Autodesk Inventor part; units mm, degrees
(part 6 of 15)
  arc A2446 (57.485, 40.2522) -> (57.485, 40.3538) centre (57.485, 40.303) ccw
  line L1082 (56.215, 40.303) -> (56.215, 43.097)
  arc A2447 (56.2658, 43.097) -> (56.1642, 43.097) centre (56.215, 43.097) ccw
  arc A2448 (56.1642, 40.303) -> (56.2658, 40.303) centre (56.215, 40.303) ccw
  line L1083 (56.215, 43.097) -> (57.485, 43.097)
  arc A2449 (57.485, 43.0462) -> (57.485, 43.1478) centre (57.485, 43.097) ccw
  arc A2450 (56.215, 43.1478) -> (56.215, 43.0462) centre (56.215, 43.097) ccw
  line L1084 (-14.55, 7.3) -> (-13.46, 7.3)
  line L1085 (59.642, 47.084) -> (59.642, 49.116)
  arc A2451 (59.6928, 49.116) -> (59.5912, 49.116) centre (59.642, 49.116) ccw
  arc A2452 (59.5912, 47.084) -> (59.6928, 47.084) centre (59.642, 47.084) ccw
  line L1086 (59.642, 49.116) -> (60.658, 49.116)
  arc A2453 (60.658, 49.0652) -> (60.658, 49.1668) centre (60.658, 49.116) ccw
  arc A2454 (59.642, 49.1668) -> (59.642, 49.0652) centre (59.642, 49.116) ccw
  line L1087 (60.658, 49.116) -> (60.658, 47.084)
  arc A2455 (60.6072, 47.084) -> (60.7088, 47.084) centre (60.658, 47.084) ccw
  arc A2456 (60.7088, 49.116) -> (60.6072, 49.116) centre (60.658, 49.116) ccw
  line L1088 (60.658, 47.084) -> (59.642, 47.084)
  arc A2457 (59.642, 47.1348) -> (59.642, 47.0332) centre (59.642, 47.084) ccw
  arc A2458 (60.658, 47.0332) -> (60.658, 47.1348) centre (60.658, 47.084) ccw
  arc A2459 (-13.46, 7.275) -> (-13.46, 7.325) centre (-13.46, 7.3) ccw
  line L1089 (52.658, 51.116) -> (52.658, 49.084)
  arc A2460 (52.6072, 49.084) -> (52.7088, 49.084) centre (52.658, 49.084) ccw
  arc A2461 (52.7088, 51.116) -> (52.6072, 51.116) centre (52.658, 51.116) ccw
  line L1090 (52.658, 49.084) -> (51.642, 49.084)
  arc A2462 (51.642, 49.1348) -> (51.642, 49.0332) centre (51.642, 49.084) ccw
  arc A2463 (52.658, 49.0332) -> (52.658, 49.1348) centre (52.658, 49.084) ccw
  line L1091 (51.642, 49.084) -> (51.642, 51.116)
  arc A2464 (51.6928, 51.116) -> (51.5912, 51.116) centre (51.642, 51.116) ccw
  arc A2465 (51.5912, 49.084) -> (51.6928, 49.084) centre (51.642, 49.084) ccw
  line L1092 (51.642, 51.116) -> (52.658, 51.116)
  arc A2466 (52.658, 51.0652) -> (52.658, 51.1668) centre (52.658, 51.116) ccw
  arc A2467 (51.642, 51.1668) -> (51.642, 51.0652) centre (51.642, 51.116) ccw
  arc A2468 (-14.55, 7.325) -> (-14.55, 7.275) centre (-14.55, 7.3) ccw
  line L1093 (46.293, 49.3892) -> (46.293, 44.4108)
  arc A2469 (46.2422, 44.4108) -> (46.3438, 44.4108) centre (46.293, 44.4108) ccw
  arc A2470 (46.3438, 49.3892) -> (46.2422, 49.3892) centre (46.293, 49.3892) ccw
  line L1094 (46.293, 44.4108) -> (44.007, 44.4108)
  arc A2471 (44.007, 44.4616) -> (44.007, 44.36) centre (44.007, 44.4108) ccw
  arc A2472 (46.293, 44.36) -> (46.293, 44.4616) centre (46.293, 44.4108) ccw
  line L1095 (44.007, 44.4108) -> (44.007, 49.3892)
  arc A2473 (44.0578, 49.3892) -> (43.9562, 49.3892) centre (44.007, 49.3892) ccw
  arc A2474 (43.9562, 44.4108) -> (44.0578, 44.4108) centre (44.007, 44.4108) ccw
  line L1096 (44.007, 49.3892) -> (46.293, 49.3892)
  arc A2475 (46.293, 49.3384) -> (46.293, 49.44) centre (46.293, 49.3892) ccw
  arc A2476 (44.007, 49.44) -> (44.007, 49.3384) centre (44.007, 49.3892) ccw
  line L1097 (-14.75, 4.1) -> (-14.75, 7.3)
  line L1098 (49.634, 46.108) -> (51.666, 46.108)
  arc A2477 (51.666, 46.0572) -> (51.666, 46.1588) centre (51.666, 46.108) ccw
  arc A2478 (49.634, 46.1588) -> (49.634, 46.0572) centre (49.634, 46.108) ccw
  line L1099 (51.666, 46.108) -> (51.666, 45.092)
  arc A2479 (51.6152, 45.092) -> (51.7168, 45.092) centre (51.666, 45.092) ccw
  arc A2480 (51.7168, 46.108) -> (51.6152, 46.108) centre (51.666, 46.108) ccw
  line L1100 (51.666, 45.092) -> (49.634, 45.092)
  arc A2481 (49.634, 45.1428) -> (49.634, 45.0412) centre (49.634, 45.092) ccw
  arc A2482 (51.666, 45.0412) -> (51.666, 45.1428) centre (51.666, 45.092) ccw
  line L1101 (49.634, 45.092) -> (49.634, 46.108)
  arc A2483 (49.6848, 46.108) -> (49.5832, 46.108) centre (49.634, 46.108) ccw
  arc A2484 (49.5832, 45.092) -> (49.6848, 45.092) centre (49.634, 45.092) ccw
  arc A2485 (-14.725, 7.3) -> (-14.775, 7.3) centre (-14.75, 7.3) ccw
  line L1102 (60.642, 47.034) -> (60.642, 49.066)
  arc A2486 (60.6928, 49.066) -> (60.5912, 49.066) centre (60.642, 49.066) ccw
  arc A2487 (60.5912, 47.034) -> (60.6928, 47.034) centre (60.642, 47.034) ccw
  line L1103 (60.642, 49.066) -> (61.658, 49.066)
  arc A2488 (61.658, 49.0152) -> (61.658, 49.1168) centre (61.658, 49.066) ccw
  arc A2489 (60.642, 49.1168) -> (60.642, 49.0152) centre (60.642, 49.066) ccw
  line L1104 (61.658, 49.066) -> (61.658, 47.034)
  arc A2490 (61.6072, 47.034) -> (61.7088, 47.034) centre (61.658, 47.034) ccw
  arc A2491 (61.7088, 49.066) -> (61.6072, 49.066) centre (61.658, 49.066) ccw
  line L1105 (61.658, 47.034) -> (60.642, 47.034)
  arc A2492 (60.642, 47.0848) -> (60.642, 46.9832) centre (60.642, 47.034) ccw
  arc A2493 (61.658, 46.9832) -> (61.658, 47.0848) centre (61.658, 47.034) ccw
  arc A2494 (-14.775, 4.1) -> (-14.725, 4.1) centre (-14.75, 4.1) ccw
  line L1106 (51.658, 51.116) -> (51.658, 49.084)
  arc A2495 (51.6072, 49.084) -> (51.7088, 49.084) centre (51.658, 49.084) ccw
  arc A2496 (51.7088, 51.116) -> (51.6072, 51.116) centre (51.658, 51.116) ccw
  line L1107 (51.658, 49.084) -> (50.642, 49.084)
  arc A2497 (50.642, 49.1348) -> (50.642, 49.0332) centre (50.642, 49.084) ccw
  arc A2498 (51.658, 49.0332) -> (51.658, 49.1348) centre (51.658, 49.084) ccw
  line L1108 (50.642, 49.084) -> (50.642, 51.116)
  arc A2499 (50.6928, 51.116) -> (50.5912, 51.116) centre (50.642, 51.116) ccw
  arc A2500 (50.5912, 49.084) -> (50.6928, 49.084) centre (50.642, 49.084) ccw
  line L1109 (50.642, 51.116) -> (51.658, 51.116)
  arc A2501 (51.658, 51.0652) -> (51.658, 51.1668) centre (51.658, 51.116) ccw
  arc A2502 (50.642, 51.1668) -> (50.642, 51.0652) centre (50.642, 51.116) ccw
  line L1110 (-14.75, 7.3) -> (-13.25, 7.3)
  line L1111 (48.585, 41.997) -> (48.585, 39.203)
  arc A2503 (48.5342, 39.203) -> (48.6358, 39.203) centre (48.585, 39.203) ccw
  arc A2504 (48.6358, 41.997) -> (48.5342, 41.997) centre (48.585, 41.997) ccw
  line L1112 (48.585, 39.203) -> (47.315, 39.203)
  arc A2505 (47.315, 39.2538) -> (47.315, 39.1522) centre (47.315, 39.203) ccw
  arc A2506 (48.585, 39.1522) -> (48.585, 39.2538) centre (48.585, 39.203) ccw
  line L1113 (47.315, 39.203) -> (47.315, 41.997)
  arc A2507 (47.3658, 41.997) -> (47.2642, 41.997) centre (47.315, 41.997) ccw
  arc A2508 (47.2642, 39.203) -> (47.3658, 39.203) centre (47.315, 39.203) ccw
  line L1114 (47.315, 41.997) -> (48.585, 41.997)
  arc A2509 (48.585, 41.9462) -> (48.585, 42.0478) centre (48.585, 41.997) ccw
  arc A2510 (47.315, 42.0478) -> (47.315, 41.9462) centre (47.315, 41.997) ccw
  arc A2511 (-13.25, 7.275) -> (-13.25, 7.325) centre (-13.25, 7.3) ccw
  line L1115 (59.642, 45.084) -> (59.642, 47.116)
  arc A2512 (59.6928, 47.116) -> (59.5912, 47.116) centre (59.642, 47.116) ccw
  arc A2513 (59.5912, 45.084) -> (59.6928, 45.084) centre (59.642, 45.084) ccw
  line L1116 (59.642, 47.116) -> (60.658, 47.116)
  arc A2514 (60.658, 47.0652) -> (60.658, 47.1668) centre (60.658, 47.116) ccw
  arc A2515 (59.642, 47.1668) -> (59.642, 47.0652) centre (59.642, 47.116) ccw
  line L1117 (60.658, 47.116) -> (60.658, 45.084)
  arc A2516 (60.6072, 45.084) -> (60.7088, 45.084) centre (60.658, 45.084) ccw
  arc A2517 (60.7088, 47.116) -> (60.6072, 47.116) centre (60.658, 47.116) ccw
  line L1118 (60.658, 45.084) -> (59.642, 45.084)
  arc A2518 (59.642, 45.1348) -> (59.642, 45.0332) centre (59.642, 45.084) ccw
  arc A2519 (60.658, 45.0332) -> (60.658, 45.1348) centre (60.658, 45.084) ccw
  arc A2520 (-14.75, 7.325) -> (-14.75, 7.275) centre (-14.75, 7.3) ccw
  line L1119 (51.642, 38.084) -> (51.642, 40.116)
  arc A2521 (51.6928, 40.116) -> (51.5912, 40.116) centre (51.642, 40.116) ccw
  arc A2522 (51.5912, 38.084) -> (51.6928, 38.084) centre (51.642, 38.084) ccw
  line L1120 (51.642, 40.116) -> (52.658, 40.116)
  arc A2523 (52.658, 40.0652) -> (52.658, 40.1668) centre (52.658, 40.116) ccw
  arc A2524 (51.642, 40.1668) -> (51.642, 40.0652) centre (51.642, 40.116) ccw
  line L1121 (52.658, 40.116) -> (52.658, 38.084)
  arc A2525 (52.6072, 38.084) -> (52.7088, 38.084) centre (52.658, 38.084) ccw
  arc A2526 (52.7088, 40.116) -> (52.6072, 40.116) centre (52.658, 40.116) ccw
  line L1122 (52.658, 38.084) -> (51.642, 38.084)
  arc A2527 (51.642, 38.1348) -> (51.642, 38.0332) centre (51.642, 38.084) ccw
  arc A2528 (52.658, 38.0332) -> (52.658, 38.1348) centre (52.658, 38.084) ccw
  line L1123 (-13.25, 7.3) -> (-13.25, 4.1)
  line L1124 (54.666, 47.092) -> (52.634, 47.092)
  arc A2529 (52.634, 47.1428) -> (52.634, 47.0412) centre (52.634, 47.092) ccw
  arc A2530 (54.666, 47.0412) -> (54.666, 47.1428) centre (54.666, 47.092) ccw
  line L1125 (52.634, 47.092) -> (52.634, 48.108)
  arc A2531 (52.6848, 48.108) -> (52.5832, 48.108) centre (52.634, 48.108) ccw
  arc A2532 (52.5832, 47.092) -> (52.6848, 47.092) centre (52.634, 47.092) ccw
  line L1126 (52.634, 48.108) -> (54.666, 48.108)
  arc A2533 (54.666, 48.0572) -> (54.666, 48.1588) centre (54.666, 48.108) ccw
  arc A2534 (52.634, 48.1588) -> (52.634, 48.0572) centre (52.634, 48.108) ccw
  line L1127 (54.666, 48.108) -> (54.666, 47.092)
  arc A2535 (54.6152, 47.092) -> (54.7168, 47.092) centre (54.666, 47.092) ccw
  arc A2536 (54.7168, 48.108) -> (54.6152, 48.108) centre (54.666, 48.108) ccw
  arc A2537 (-13.275, 4.1) -> (-13.225, 4.1) centre (-13.25, 4.1) ccw
  line L1128 (49.634, 42.108) -> (51.666, 42.108)
  arc A2538 (51.666, 42.0572) -> (51.666, 42.1588) centre (51.666, 42.108) ccw
  arc A2539 (49.634, 42.1588) -> (49.634, 42.0572) centre (49.634, 42.108) ccw
  line L1129 (51.666, 42.108) -> (51.666, 41.092)
  arc A2540 (51.6152, 41.092) -> (51.7168, 41.092) centre (51.666, 41.092) ccw
  arc A2541 (51.7168, 42.108) -> (51.6152, 42.108) centre (51.666, 42.108) ccw
  line L1130 (51.666, 41.092) -> (49.634, 41.092)
  arc A2542 (49.634, 41.1428) -> (49.634, 41.0412) centre (49.634, 41.092) ccw
  arc A2543 (51.666, 41.0412) -> (51.666, 41.1428) centre (51.666, 41.092) ccw
  line L1131 (49.634, 41.092) -> (49.634, 42.108)
  arc A2544 (49.6848, 42.108) -> (49.5832, 42.108) centre (49.634, 42.108) ccw
  arc A2545 (49.5832, 41.092) -> (49.6848, 41.092) centre (49.634, 41.092) ccw
  arc A2546 (-13.225, 7.3) -> (-13.275, 7.3) centre (-13.25, 7.3) ccw
  line L1132 (60.642, 45.084) -> (60.642, 47.116)
  arc A2547 (60.6928, 47.116) -> (60.5912, 47.116) centre (60.642, 47.116) ccw
  arc A2548 (60.5912, 45.084) -> (60.6928, 45.084) centre (60.642, 45.084) ccw
  line L1133 (60.642, 47.116) -> (61.658, 47.116)
  arc A2549 (61.658, 47.0652) -> (61.658, 47.1668) centre (61.658, 47.116) ccw
  arc A2550 (60.642, 47.1668) -> (60.642, 47.0652) centre (60.642, 47.116) ccw
  line L1134 (61.658, 47.116) -> (61.658, 45.084)
  arc A2551 (61.6072, 45.084) -> (61.7088, 45.084) centre (61.658, 45.084) ccw
  arc A2552 (61.7088, 47.116) -> (61.6072, 47.116) centre (61.658, 47.116) ccw
  line L1135 (61.658, 45.084) -> (60.642, 45.084)
  arc A2553 (60.642, 45.1348) -> (60.642, 45.0332) centre (60.642, 45.084) ccw
  arc A2554 (61.658, 45.0332) -> (61.658, 45.1348) centre (61.658, 45.084) ccw
  line L1136 (-13.25, 4.1) -> (-14.75, 4.1)
  line L1137 (52.642, 38.084) -> (52.642, 40.116)
  arc A2555 (52.6928, 40.116) -> (52.5912, 40.116) centre (52.642, 40.116) ccw
  arc A2556 (52.5912, 38.084) -> (52.6928, 38.084) centre (52.642, 38.084) ccw
  line L1138 (52.642, 40.116) -> (53.658, 40.116)
  arc A2557 (53.658, 40.0652) -> (53.658, 40.1668) centre (53.658, 40.116) ccw
  arc A2558 (52.642, 40.1668) -> (52.642, 40.0652) centre (52.642, 40.116) ccw
  line L1139 (53.658, 40.116) -> (53.658, 38.084)
  arc A2559 (53.6072, 38.084) -> (53.7088, 38.084) centre (53.658, 38.084) ccw
  arc A2560 (53.7088, 40.116) -> (53.6072, 40.116) centre (53.658, 40.116) ccw
  line L1140 (53.658, 38.084) -> (52.642, 38.084)
  arc A2561 (52.642, 38.1348) -> (52.642, 38.0332) centre (52.642, 38.084) ccw
  arc A2562 (53.658, 38.0332) -> (53.658, 38.1348) centre (53.658, 38.084) ccw
  arc A2563 (-14.75, 4.125) -> (-14.75, 4.075) centre (-14.75, 4.1) ccw
  line L1141 (54.666, 41.092) -> (52.634, 41.092)
  arc A2564 (52.634, 41.1428) -> (52.634, 41.0412) centre (52.634, 41.092) ccw
  arc A2565 (54.666, 41.0412) -> (54.666, 41.1428) centre (54.666, 41.092) ccw
  line L1142 (52.634, 41.092) -> (52.634, 42.108)
  arc A2566 (52.6848, 42.108) -> (52.5832, 42.108) centre (52.634, 42.108) ccw
  arc A2567 (52.5832, 41.092) -> (52.6848, 41.092) centre (52.634, 41.092) ccw
  line L1143 (52.634, 42.108) -> (54.666, 42.108)
  arc A2568 (54.666, 42.0572) -> (54.666, 42.1588) centre (54.666, 42.108) ccw
  arc A2569 (52.634, 42.1588) -> (52.634, 42.0572) centre (52.634, 42.108) ccw
  line L1144 (54.666, 42.108) -> (54.666, 41.092)
  arc A2570 (54.6152, 41.092) -> (54.7168, 41.092) centre (54.666, 41.092) ccw
  arc A2571 (54.7168, 42.108) -> (54.6152, 42.108) centre (54.666, 42.108) ccw
  arc A2572 (-13.25, 4.075) -> (-13.25, 4.125) centre (-13.25, 4.1) ccw
  line L1145 (57.634, 48.108) -> (59.666, 48.108)
  arc A2573 (59.666, 48.0572) -> (59.666, 48.1588) centre (59.666, 48.108) ccw
  arc A2574 (57.634, 48.1588) -> (57.634, 48.0572) centre (57.634, 48.108) ccw
  line L1146 (59.666, 48.108) -> (59.666, 47.092)
  arc A2575 (59.6152, 47.092) -> (59.7168, 47.092) centre (59.666, 47.092) ccw
  arc A2576 (59.7168, 48.108) -> (59.6152, 48.108) centre (59.666, 48.108) ccw
  line L1147 (59.666, 47.092) -> (57.634, 47.092)
  arc A2577 (57.634, 47.1428) -> (57.634, 47.0412) centre (57.634, 47.092) ccw
  arc A2578 (59.666, 47.0412) -> (59.666, 47.1428) centre (59.666, 47.092) ccw
  line L1148 (57.634, 47.092) -> (57.634, 48.108)
  arc A2579 (57.6848, 48.108) -> (57.5832, 48.108) centre (57.634, 48.108) ccw
  arc A2580 (57.5832, 47.092) -> (57.6848, 47.092) centre (57.634, 47.092) ccw
  arc A2581 (-14.4, 4.435) -> (-14.4, 4.585) centre (-14.4, 4.51) ccw
  line L1149 (54.634, 49.108) -> (56.666, 49.108)
  arc A2582 (56.666, 49.0572) -> (56.666, 49.1588) centre (56.666, 49.108) ccw
  arc A2583 (54.634, 49.1588) -> (54.634, 49.0572) centre (54.634, 49.108) ccw
  line L1150 (56.666, 49.108) -> (56.666, 48.092)
  arc A2584 (56.6152, 48.092) -> (56.7168, 48.092) centre (56.666, 48.092) ccw
  arc A2585 (56.7168, 49.108) -> (56.6152, 49.108) centre (56.666, 49.108) ccw
  line L1151 (56.666, 48.092) -> (54.634, 48.092)
  arc A2586 (54.634, 48.1428) -> (54.634, 48.0412) centre (54.634, 48.092) ccw
  arc A2587 (56.666, 48.0412) -> (56.666, 48.1428) centre (56.666, 48.092) ccw
  line L1152 (54.634, 48.092) -> (54.634, 49.108)
  arc A2588 (54.6848, 49.108) -> (54.5832, 49.108) centre (54.634, 49.108) ccw
  arc A2589 (54.5832, 48.092) -> (54.6848, 48.092) centre (54.634, 48.092) ccw
  arc A2590 (-14.4, 4.585) -> (-14.4, 4.435) centre (-14.4, 4.51) ccw
  line L1153 (54.642, 38.084) -> (54.642, 40.116)
  arc A2591 (54.6928, 40.116) -> (54.5912, 40.116) centre (54.642, 40.116) ccw
  arc A2592 (54.5912, 38.084) -> (54.6928, 38.084) centre (54.642, 38.084) ccw
  line L1154 (54.642, 40.116) -> (55.658, 40.116)
  arc A2593 (55.658, 40.0652) -> (55.658, 40.1668) centre (55.658, 40.116) ccw
  arc A2594 (54.642, 40.1668) -> (54.642, 40.0652) centre (54.642, 40.116) ccw
  line L1155 (55.658, 40.116) -> (55.658, 38.084)
  arc A2595 (55.6072, 38.084) -> (55.7088, 38.084) centre (55.658, 38.084) ccw
  arc A2596 (55.7088, 40.116) -> (55.6072, 40.116) centre (55.658, 40.116) ccw
  line L1156 (55.658, 38.084) -> (54.642, 38.084)
  arc A2597 (54.642, 38.1348) -> (54.642, 38.0332) centre (54.642, 38.084) ccw
  arc A2598 (55.658, 38.0332) -> (55.658, 38.1348) centre (55.658, 38.084) ccw
  line L1157 (60.5, 37.4) -> (60.5, 36.6)
  line L1158 (56.642, 38.084) -> (56.642, 40.116)
  arc A2599 (56.6928, 40.116) -> (56.5912, 40.116) centre (56.642, 40.116) ccw
  arc A2600 (56.5912, 38.084) -> (56.6928, 38.084) centre (56.642, 38.084) ccw
  line L1159 (56.642, 40.116) -> (57.658, 40.116)
  arc A2601 (57.658, 40.0652) -> (57.658, 40.1668) centre (57.658, 40.116) ccw
  arc A2602 (56.642, 40.1668) -> (56.642, 40.0652) centre (56.642, 40.116) ccw
  line L1160 (57.658, 40.116) -> (57.658, 38.084)
  arc A2603 (57.6072, 38.084) -> (57.7088, 38.084) centre (57.658, 38.084) ccw
  arc A2604 (57.7088, 40.116) -> (57.6072, 40.116) centre (57.658, 40.116) ccw
  line L1161 (57.658, 38.084) -> (56.642, 38.084)
  arc A2605 (56.642, 38.1348) -> (56.642, 38.0332) centre (56.642, 38.084) ccw
  arc A2606 (57.658, 38.0332) -> (57.658, 38.1348) centre (57.658, 38.084) ccw
  arc A2607 (60.4683, 36.6) -> (60.5317, 36.6) centre (60.5, 36.6) ccw
  line L1162 (57.634, 42.108) -> (59.666, 42.108)
  arc A2608 (59.666, 42.0572) -> (59.666, 42.1588) centre (59.666, 42.108) ccw
  arc A2609 (57.634, 42.1588) -> (57.634, 42.0572) centre (57.634, 42.108) ccw
  line L1163 (59.666, 42.108) -> (59.666, 41.092)
  arc A2610 (59.6152, 41.092) -> (59.7168, 41.092) centre (59.666, 41.092) ccw
  arc A2611 (59.7168, 42.108) -> (59.6152, 42.108) centre (59.666, 42.108) ccw
  line L1164 (59.666, 41.092) -> (57.634, 41.092)
  arc A2612 (57.634, 41.1428) -> (57.634, 41.0412) centre (57.634, 41.092) ccw
  arc A2613 (59.666, 41.0412) -> (59.666, 41.1428) centre (59.666, 41.092) ccw
  line L1165 (57.634, 41.092) -> (57.634, 42.108)
  arc A2614 (57.6848, 42.108) -> (57.5832, 42.108) centre (57.634, 42.108) ccw
  arc A2615 (57.5832, 41.092) -> (57.6848, 41.092) centre (57.634, 41.092) ccw
  arc A2616 (60.5317, 37.4) -> (60.4683, 37.4) centre (60.5, 37.4) ccw
  line L1166 (54.634, 48.108) -> (56.666, 48.108)
  arc A2617 (56.666, 48.0572) -> (56.666, 48.1588) centre (56.666, 48.108) ccw
  arc A2618 (54.634, 48.1588) -> (54.634, 48.0572) centre (54.634, 48.108) ccw
  line L1167 (56.666, 48.108) -> (56.666, 47.092)
  arc A2619 (56.6152, 47.092) -> (56.7168, 47.092) centre (56.666, 47.092) ccw
  arc A2620 (56.7168, 48.108) -> (56.6152, 48.108) centre (56.666, 48.108) ccw
  line L1168 (56.666, 47.092) -> (54.634, 47.092)
  arc A2621 (54.634, 47.1428) -> (54.634, 47.0412) centre (54.634, 47.092) ccw
  arc A2622 (56.666, 47.0412) -> (56.666, 47.1428) centre (56.666, 47.092) ccw
  line L1169 (54.634, 47.092) -> (54.634, 48.108)
  arc A2623 (54.6848, 48.108) -> (54.5832, 48.108) centre (54.634, 48.108) ccw
  arc A2624 (54.5832, 47.092) -> (54.6848, 47.092) centre (54.634, 47.092) ccw
  line L1170 (63, 36.6) -> (63, 37.4)
  line L1171 (55.666, 37.092) -> (53.634, 37.092)
  arc A2625 (53.634, 37.1428) -> (53.634, 37.0412) centre (53.634, 37.092) ccw
  arc A2626 (55.666, 37.0412) -> (55.666, 37.1428) centre (55.666, 37.092) ccw
  line L1172 (53.634, 37.092) -> (53.634, 38.108)
  arc A2627 (53.6848, 38.108) -> (53.5832, 38.108) centre (53.634, 38.108) ccw
  arc A2628 (53.5832, 37.092) -> (53.6848, 37.092) centre (53.634, 37.092) ccw
  line L1173 (53.634, 38.108) -> (55.666, 38.108)
  arc A2629 (55.666, 38.0572) -> (55.666, 38.1588) centre (55.666, 38.108) ccw
  arc A2630 (53.634, 38.1588) -> (53.634, 38.0572) centre (53.634, 38.108) ccw
  line L1174 (55.666, 38.108) -> (55.666, 37.092)
  arc A2631 (55.6152, 37.092) -> (55.7168, 37.092) centre (55.666, 37.092) ccw
  arc A2632 (55.7168, 38.108) -> (55.6152, 38.108) centre (55.666, 38.108) ccw
  arc A2633 (63.0317, 37.4) -> (62.9683, 37.4) centre (63, 37.4) ccw
  line L1175 (55.642, 38.084) -> (55.642, 40.116)
  arc A2634 (55.6928, 40.116) -> (55.5912, 40.116) centre (55.642, 40.116) ccw
  arc A2635 (55.5912, 38.084) -> (55.6928, 38.084) centre (55.642, 38.084) ccw
  line L1176 (55.642, 40.116) -> (56.658, 40.116)
  arc A2636 (56.658, 40.0652) -> (56.658, 40.1668) centre (56.658, 40.116) ccw
  arc A2637 (55.642, 40.1668) -> (55.642, 40.0652) centre (55.642, 40.116) ccw
  line L1177 (56.658, 40.116) -> (56.658, 38.084)
  arc A2638 (56.6072, 38.084) -> (56.7088, 38.084) centre (56.658, 38.084) ccw
  arc A2639 (56.7088, 40.116) -> (56.6072, 40.116) centre (56.658, 40.116) ccw
  line L1178 (56.658, 38.084) -> (55.642, 38.084)
  arc A2640 (55.642, 38.1348) -> (55.642, 38.0332) centre (55.642, 38.084) ccw
  arc A2641 (56.658, 38.0332) -> (56.658, 38.1348) centre (56.658, 38.084) ccw
  arc A2642 (62.9683, 36.6) -> (63.0317, 36.6) centre (63, 36.6) ccw
  line L1179 (49.634, 40.108) -> (51.666, 40.108)
  arc A2643 (51.666, 40.0572) -> (51.666, 40.1588) centre (51.666, 40.108) ccw
  arc A2644 (49.634, 40.1588) -> (49.634, 40.0572) centre (49.634, 40.108) ccw
  line L1180 (51.666, 40.108) -> (51.666, 39.092)
  arc A2645 (51.6152, 39.092) -> (51.7168, 39.092) centre (51.666, 39.092) ccw
  arc A2646 (51.7168, 40.108) -> (51.6152, 40.108) centre (51.666, 40.108) ccw
  line L1181 (51.666, 39.092) -> (49.634, 39.092)
  arc A2647 (49.634, 39.1428) -> (49.634, 39.0412) centre (49.634, 39.092) ccw
  arc A2648 (51.666, 39.0412) -> (51.666, 39.1428) centre (51.666, 39.092) ccw
  line L1182 (49.634, 39.092) -> (49.634, 40.108)
  arc A2649 (49.6848, 40.108) -> (49.5832, 40.108) centre (49.634, 40.108) ccw
  arc A2650 (49.5832, 39.092) -> (49.6848, 39.092) centre (49.634, 39.092) ccw
  line L1183 (61.45, 35.4) -> (62.05, 35.4)
  line L1184 (61.985, 42.997) -> (61.985, 40.203)
  arc A2651 (61.9342, 40.203) -> (62.0358, 40.203) centre (61.985, 40.203) ccw
  arc A2652 (62.0358, 42.997) -> (61.9342, 42.997) centre (61.985, 42.997) ccw
  line L1185 (61.985, 40.203) -> (60.715, 40.203)
  arc A2653 (60.715, 40.2538) -> (60.715, 40.1522) centre (60.715, 40.203) ccw
  arc A2654 (61.985, 40.1522) -> (61.985, 40.2538) centre (61.985, 40.203) ccw
  line L1186 (60.715, 40.203) -> (60.715, 42.997)
  arc A2655 (60.7658, 42.997) -> (60.6642, 42.997) centre (60.715, 42.997) ccw
  arc A2656 (60.6642, 40.203) -> (60.7658, 40.203) centre (60.715, 40.203) ccw
  line L1187 (60.715, 42.997) -> (61.985, 42.997)
  arc A2657 (61.985, 42.9462) -> (61.985, 43.0478) centre (61.985, 42.997) ccw
  arc A2658 (60.715, 43.0478) -> (60.715, 42.9462) centre (60.715, 42.997) ccw
  arc A2659 (62.05, 35.3683) -> (62.05, 35.4317) centre (62.05, 35.4) ccw
  line L1188 (61.658, 51.116) -> (61.658, 49.084)
  arc A2660 (61.6072, 49.084) -> (61.7088, 49.084) centre (61.658, 49.084) ccw
  arc A2661 (61.7088, 51.116) -> (61.6072, 51.116) centre (61.658, 51.116) ccw
  line L1189 (61.658, 49.084) -> (60.642, 49.084)
  arc A2662 (60.642, 49.1348) -> (60.642, 49.0332) centre (60.642, 49.084) ccw
  arc A2663 (61.658, 49.0332) -> (61.658, 49.1348) centre (61.658, 49.084) ccw
  line L1190 (60.642, 49.084) -> (60.642, 51.116)
  arc A2664 (60.6928, 51.116) -> (60.5912, 51.116) centre (60.642, 51.116) ccw
  arc A2665 (60.5912, 49.084) -> (60.6928, 49.084) centre (60.642, 49.084) ccw
  line L1191 (60.642, 51.116) -> (61.658, 51.116)
  arc A2666 (61.658, 51.0652) -> (61.658, 51.1668) centre (61.658, 51.116) ccw
  arc A2667 (60.642, 51.1668) -> (60.642, 51.0652) centre (60.642, 51.116) ccw
  arc A2668 (61.45, 35.4317) -> (61.45, 35.3683) centre (61.45, 35.4) ccw
  line L1192 (56.085, 43.097) -> (56.085, 40.303)
  arc A2669 (56.0342, 40.303) -> (56.1358, 40.303) centre (56.085, 40.303) ccw
  arc A2670 (56.1358, 43.097) -> (56.0342, 43.097) centre (56.085, 43.097) ccw
  line L1193 (56.085, 40.303) -> (54.815, 40.303)
  arc A2671 (54.815, 40.3538) -> (54.815, 40.2522) centre (54.815, 40.303) ccw
  arc A2672 (56.085, 40.2522) -> (56.085, 40.3538) centre (56.085, 40.303) ccw
  line L1194 (54.815, 40.303) -> (54.815, 43.097)
  arc A2673 (54.8658, 43.097) -> (54.7642, 43.097) centre (54.815, 43.097) ccw
  arc A2674 (54.7642, 40.303) -> (54.8658, 40.303) centre (54.815, 40.303) ccw
  line L1195 (54.815, 43.097) -> (56.085, 43.097)
  arc A2675 (56.085, 43.0462) -> (56.085, 43.1478) centre (56.085, 43.097) ccw
  arc A2676 (54.815, 43.1478) -> (54.815, 43.0462) centre (54.815, 43.097) ccw
  line L1196 (62.05, 38.6) -> (61.45, 38.6)
  line L1197 (49.634, 41.108) -> (51.666, 41.108)
  arc A2677 (51.666, 41.0572) -> (51.666, 41.1588) centre (51.666, 41.108) ccw
  arc A2678 (49.634, 41.1588) -> (49.634, 41.0572) centre (49.634, 41.108) ccw
  line L1198 (51.666, 41.108) -> (51.666, 40.092)
  arc A2679 (51.6152, 40.092) -> (51.7168, 40.092) centre (51.666, 40.092) ccw
  arc A2680 (51.7168, 41.108) -> (51.6152, 41.108) centre (51.666, 41.108) ccw
  line L1199 (51.666, 40.092) -> (49.634, 40.092)
  arc A2681 (49.634, 40.1428) -> (49.634, 40.0412) centre (49.634, 40.092) ccw
  arc A2682 (51.666, 40.0412) -> (51.666, 40.1428) centre (51.666, 40.092) ccw
  line L1200 (49.634, 40.092) -> (49.634, 41.108)
  arc A2683 (49.6848, 41.108) -> (49.5832, 41.108) centre (49.634, 41.108) ccw
  arc A2684 (49.5832, 40.092) -> (49.6848, 40.092) centre (49.634, 40.092) ccw
  arc A2685 (61.45, 38.6318) -> (61.45, 38.5683) centre (61.45, 38.6) ccw
  line L1201 (60.658, 51.116) -> (60.658, 49.084)
  arc A2686 (60.6072, 49.084) -> (60.7088, 49.084) centre (60.658, 49.084) ccw
  arc A2687 (60.7088, 51.116) -> (60.6072, 51.116) centre (60.658, 51.116) ccw
  line L1202 (60.658, 49.084) -> (59.642, 49.084)
  arc A2688 (59.642, 49.1348) -> (59.642, 49.0332) centre (59.642, 49.084) ccw
  arc A2689 (60.658, 49.0332) -> (60.658, 49.1348) centre (60.658, 49.084) ccw
  line L1203 (59.642, 49.084) -> (59.642, 51.116)
  arc A2690 (59.6928, 51.116) -> (59.5912, 51.116) centre (59.642, 51.116) ccw
  arc A2691 (59.5912, 49.084) -> (59.6928, 49.084) centre (59.642, 49.084) ccw
  line L1204 (59.642, 51.116) -> (60.658, 51.116)
  arc A2692 (60.658, 51.0652) -> (60.658, 51.1668) centre (60.658, 51.116) ccw
  arc A2693 (59.642, 51.1668) -> (59.642, 51.0652) centre (59.642, 51.116) ccw
  arc A2694 (62.05, 38.5683) -> (62.05, 38.6318) centre (62.05, 38.6) ccw
  line L1205 (50.658, 45.116) -> (50.658, 43.084)
  arc A2695 (50.6072, 43.084) -> (50.7088, 43.084) centre (50.658, 43.084) ccw
  arc A2696 (50.7088, 45.116) -> (50.6072, 45.116) centre (50.658, 45.116) ccw
  line L1206 (50.658, 43.084) -> (49.642, 43.084)
  arc A2697 (49.642, 43.1348) -> (49.642, 43.0332) centre (49.642, 43.084) ccw
  arc A2698 (50.658, 43.0332) -> (50.658, 43.1348) centre (50.658, 43.084) ccw
  line L1207 (49.642, 43.084) -> (49.642, 45.116)
  arc A2699 (49.6928, 45.116) -> (49.5912, 45.116) centre (49.642, 45.116) ccw
  arc A2700 (49.5912, 43.084) -> (49.6928, 43.084) centre (49.642, 43.084) ccw
  line L1208 (49.642, 45.116) -> (50.658, 45.116)
  arc A2701 (50.658, 45.0652) -> (50.658, 45.1668) centre (50.658, 45.116) ccw
  arc A2702 (49.642, 45.1668) -> (49.642, 45.0652) centre (49.642, 45.116) ccw
  arc A2703 (62.4, 36.0293) -> (62.4, 36.1707) centre (62.4, 36.1) ccw
  line L1209 (53.658, 51.116) -> (53.658, 49.084)
  arc A2704 (53.6072, 49.084) -> (53.7088, 49.084) centre (53.658, 49.084) ccw
  arc A2705 (53.7088, 51.116) -> (53.6072, 51.116) centre (53.658, 51.116) ccw
  line L1210 (53.658, 49.084) -> (52.642, 49.084)
  arc A2706 (52.642, 49.1348) -> (52.642, 49.0332) centre (52.642, 49.084) ccw
  arc A2707 (53.658, 49.0332) -> (53.658, 49.1348) centre (53.658, 49.084) ccw
  line L1211 (52.642, 49.084) -> (52.642, 51.116)
  arc A2708 (52.6928, 51.116) -> (52.5912, 51.116) centre (52.642, 51.116) ccw
  arc A2709 (52.5912, 49.084) -> (52.6928, 49.084) centre (52.642, 49.084) ccw
  line L1212 (52.642, 51.116) -> (53.658, 51.116)
  arc A2710 (53.658, 51.0652) -> (53.658, 51.1668) centre (53.658, 51.116) ccw
  arc A2711 (52.642, 51.1668) -> (52.642, 51.0652) centre (52.642, 51.116) ccw
  arc A2712 (62.4, 36.1707) -> (62.4, 36.0293) centre (62.4, 36.1) ccw
  line L1213 (49.634, 49.108) -> (51.666, 49.108)
  arc A2713 (51.666, 49.0572) -> (51.666, 49.1588) centre (51.666, 49.108) ccw
  arc A2714 (49.634, 49.1588) -> (49.634, 49.0572) centre (49.634, 49.108) ccw
  line L1214 (51.666, 49.108) -> (51.666, 48.092)
  arc A2715 (51.6152, 48.092) -> (51.7168, 48.092) centre (51.666, 48.092) ccw
  arc A2716 (51.7168, 49.108) -> (51.6152, 49.108) centre (51.666, 49.108) ccw
  line L1215 (51.666, 48.092) -> (49.634, 48.092)
  arc A2717 (49.634, 48.1428) -> (49.634, 48.0412) centre (49.634, 48.092) ccw
  arc A2718 (51.666, 48.0412) -> (51.666, 48.1428) centre (51.666, 48.092) ccw
  line L1216 (49.634, 48.092) -> (49.634, 49.108)
  arc A2719 (49.6848, 49.108) -> (49.5832, 49.108) centre (49.634, 49.108) ccw
  arc A2720 (49.5832, 48.092) -> (49.6848, 48.092) centre (49.634, 48.092) ccw
  line L1217 (5.25, 34.15) -> (5.25, 37.25)
  line L1218 (53.642, 38.084) -> (53.642, 40.116)
  arc A2721 (53.6928, 40.116) -> (53.5912, 40.116) centre (53.642, 40.116) ccw
  arc A2722 (53.5912, 38.084) -> (53.6928, 38.084) centre (53.642, 38.084) ccw
  line L1219 (53.642, 40.116) -> (54.658, 40.116)
  arc A2723 (54.658, 40.0652) -> (54.658, 40.1668) centre (54.658, 40.116) ccw
  arc A2724 (53.642, 40.1668) -> (53.642, 40.0652) centre (53.642, 40.116) ccw
  line L1220 (54.658, 40.116) -> (54.658, 38.084)
  arc A2725 (54.6072, 38.084) -> (54.7088, 38.084) centre (54.658, 38.084) ccw
  arc A2726 (54.7088, 40.116) -> (54.6072, 40.116) centre (54.658, 40.116) ccw
  line L1221 (54.658, 38.084) -> (53.642, 38.084)
  arc A2727 (53.642, 38.1348) -> (53.642, 38.0332) centre (53.642, 38.084) ccw
  arc A2728 (54.658, 38.0332) -> (54.658, 38.1348) centre (54.658, 38.084) ccw
  arc A2729 (5.2818, 37.25) -> (5.2183, 37.25) centre (5.25, 37.25) ccw
  line L1222 (56.215, 43.103) -> (56.215, 45.897)
  arc A2730 (56.2658, 45.897) -> (56.1642, 45.897) centre (56.215, 45.897) ccw
  arc A2731 (56.1642, 43.103) -> (56.2658, 43.103) centre (56.215, 43.103) ccw
  line L1223 (56.215, 45.897) -> (57.485, 45.897)
  arc A2732 (57.485, 45.8462) -> (57.485, 45.9478) centre (57.485, 45.897) ccw
  arc A2733 (56.215, 45.9478) -> (56.215, 45.8462) centre (56.215, 45.897) ccw
  line L1224 (57.485, 45.897) -> (57.485, 43.103)
  arc A2734 (57.4342, 43.103) -> (57.5358, 43.103) centre (57.485, 43.103) ccw
  arc A2735 (57.5358, 45.897) -> (57.4342, 45.897) centre (57.485, 45.897) ccw
  line L1225 (57.485, 43.103) -> (56.215, 43.103)
  arc A2736 (56.215, 43.1538) -> (56.215, 43.0522) centre (56.215, 43.103) ccw
  arc A2737 (57.485, 43.0522) -> (57.485, 43.1538) centre (57.485, 43.103) ccw
  arc A2738 (5.2183, 34.15) -> (5.2818, 34.15) centre (5.25, 34.15) ccw
  line L1226 (57.634, 45.108) -> (59.666, 45.108)
  arc A2739 (59.666, 45.0572) -> (59.666, 45.1588) centre (59.666, 45.108) ccw
  arc A2740 (57.634, 45.1588) -> (57.634, 45.0572) centre (57.634, 45.108) ccw
  line L1227 (59.666, 45.108) -> (59.666, 44.092)
  arc A2741 (59.6152, 44.092) -> (59.7168, 44.092) centre (59.666, 44.092) ccw
  arc A2742 (59.7168, 45.108) -> (59.6152, 45.108) centre (59.666, 45.108) ccw
  line L1228 (59.666, 44.092) -> (57.634, 44.092)
  arc A2743 (57.634, 44.1428) -> (57.634, 44.0412) centre (57.634, 44.092) ccw
  arc A2744 (59.666, 44.0412) -> (59.666, 44.1428) centre (59.666, 44.092) ccw
  line L1229 (57.634, 44.092) -> (57.634, 45.108)
  arc A2745 (57.6848, 45.108) -> (57.5832, 45.108) centre (57.634, 45.108) ccw
  arc A2746 (57.5832, 44.092) -> (57.6848, 44.092) centre (57.634, 44.092) ccw
  line L1230 (5.25, 37.25) -> (7.75, 37.25)
  line L1231 (49.634, 48.108) -> (51.666, 48.108)
  arc A2747 (51.666, 48.0572) -> (51.666, 48.1588) centre (51.666, 48.108) ccw
  arc A2748 (49.634, 48.1588) -> (49.634, 48.0572) centre (49.634, 48.108) ccw
  line L1232 (51.666, 48.108) -> (51.666, 47.092)
  arc A2749 (51.6152, 47.092) -> (51.7168, 47.092) centre (51.666, 47.092) ccw
  arc A2750 (51.7168, 48.108) -> (51.6152, 48.108) centre (51.666, 48.108) ccw
  line L1233 (51.666, 47.092) -> (49.634, 47.092)
  arc A2751 (49.634, 47.1428) -> (49.634, 47.0412) centre (49.634, 47.092) ccw
  arc A2752 (51.666, 47.0412) -> (51.666, 47.1428) centre (51.666, 47.092) ccw
  line L1234 (49.634, 47.092) -> (49.634, 48.108)
  arc A2753 (49.6848, 48.108) -> (49.5832, 48.108) centre (49.634, 48.108) ccw
  arc A2754 (49.5832, 47.092) -> (49.6848, 47.092) centre (49.634, 47.092) ccw
  arc A2755 (7.75, 37.2183) -> (7.75, 37.2817) centre (7.75, 37.25) ccw
  line L1235 (57.642, 38.084) -> (57.642, 40.116)
  arc A2756 (57.6928, 40.116) -> (57.5912, 40.116) centre (57.642, 40.116) ccw
  arc A2757 (57.5912, 38.084) -> (57.6928, 38.084) centre (57.642, 38.084) ccw
  line L1236 (57.642, 40.116) -> (58.658, 40.116)
  arc A2758 (58.658, 40.0652) -> (58.658, 40.1668) centre (58.658, 40.116) ccw
  arc A2759 (57.642, 40.1668) -> (57.642, 40.0652) centre (57.642, 40.116) ccw
  line L1237 (58.658, 40.116) -> (58.658, 38.084)
  arc A2760 (58.6072, 38.084) -> (58.7088, 38.084) centre (58.658, 38.084) ccw
  arc A2761 (58.7088, 40.116) -> (58.6072, 40.116) centre (58.658, 40.116) ccw
  line L1238 (58.658, 38.084) -> (57.642, 38.084)
  arc A2762 (57.642, 38.1348) -> (57.642, 38.0332) centre (57.642, 38.084) ccw
  arc A2763 (58.658, 38.0332) -> (58.658, 38.1348) centre (58.658, 38.084) ccw
  arc A2764 (5.25, 37.2817) -> (5.25, 37.2183) centre (5.25, 37.25) ccw
  line L1239 (51.658, 45.116) -> (51.658, 43.084)
  arc A2765 (51.6072, 43.084) -> (51.7088, 43.084) centre (51.658, 43.084) ccw
  arc A2766 (51.7088, 45.116) -> (51.6072, 45.116) centre (51.658, 45.116) ccw
  line L1240 (51.658, 43.084) -> (50.642, 43.084)
  arc A2767 (50.642, 43.1348) -> (50.642, 43.0332) centre (50.642, 43.084) ccw
  arc A2768 (51.658, 43.0332) -> (51.658, 43.1348) centre (51.658, 43.084) ccw
  line L1241 (50.642, 43.084) -> (50.642, 45.116)
  arc A2769 (50.6928, 45.116) -> (50.5912, 45.116) centre (50.642, 45.116) ccw
  arc A2770 (50.5912, 43.084) -> (50.6928, 43.084) centre (50.642, 43.084) ccw
  line L1242 (50.642, 45.116) -> (51.658, 45.116)
  arc A2771 (51.658, 45.0652) -> (51.658, 45.1668) centre (51.658, 45.116) ccw
  arc A2772 (50.642, 45.1668) -> (50.642, 45.0652) centre (50.642, 45.116) ccw
  line L1243 (7.75, 37.25) -> (7.75, 34.15)
  line L1244 (54.642, 45.084) -> (54.642, 47.116)
  arc A2773 (54.6928, 47.116) -> (54.5912, 47.116) centre (54.642, 47.116) ccw
  arc A2774 (54.5912, 45.084) -> (54.6928, 45.084) centre (54.642, 45.084) ccw
  line L1245 (54.642, 47.116) -> (55.658, 47.116)
  arc A2775 (55.658, 47.0652) -> (55.658, 47.1668) centre (55.658, 47.116) ccw
  arc A2776 (54.642, 47.1668) -> (54.642, 47.0652) centre (54.642, 47.116) ccw
  line L1246 (55.658, 47.116) -> (55.658, 45.084)
  arc A2777 (55.6072, 45.084) -> (55.7088, 45.084) centre (55.658, 45.084) ccw
  arc A2778 (55.7088, 47.116) -> (55.6072, 47.116) centre (55.658, 47.116) ccw
  line L1247 (55.658, 45.084) -> (54.642, 45.084)
  arc A2779 (54.642, 45.1348) -> (54.642, 45.0332) centre (54.642, 45.084) ccw
  arc A2780 (55.658, 45.0332) -> (55.658, 45.1348) centre (55.658, 45.084) ccw
  arc A2781 (7.7183, 34.15) -> (7.7818, 34.15) centre (7.75, 34.15) ccw
  line L1248 (59.658, 51.116) -> (59.658, 49.084)
  arc A2782 (59.6072, 49.084) -> (59.7088, 49.084) centre (59.658, 49.084) ccw
  arc A2783 (59.7088, 51.116) -> (59.6072, 51.116) centre (59.658, 51.116) ccw
  line L1249 (59.658, 49.084) -> (58.642, 49.084)
  arc A2784 (58.642, 49.1348) -> (58.642, 49.0332) centre (58.642, 49.084) ccw
  arc A2785 (59.658, 49.0332) -> (59.658, 49.1348) centre (59.658, 49.084) ccw
  line L1250 (58.642, 49.084) -> (58.642, 51.116)
  arc A2786 (58.6928, 51.116) -> (58.5912, 51.116) centre (58.642, 51.116) ccw
  arc A2787 (58.5912, 49.084) -> (58.6928, 49.084) centre (58.642, 49.084) ccw
  line L1251 (58.642, 51.116) -> (59.658, 51.116)
  arc A2788 (59.658, 51.0652) -> (59.658, 51.1668) centre (59.658, 51.116) ccw
  arc A2789 (58.642, 51.1668) -> (58.642, 51.0652) centre (58.642, 51.116) ccw
  arc A2790 (7.7818, 37.25) -> (7.7183, 37.25) centre (7.75, 37.25) ccw
  line L1252 (54.666, 46.092) -> (52.634, 46.092)
  arc A2791 (52.634, 46.1428) -> (52.634, 46.0412) centre (52.634, 46.092) ccw
  arc A2792 (54.666, 46.0412) -> (54.666, 46.1428) centre (54.666, 46.092) ccw
  line L1253 (52.634, 46.092) -> (52.634, 47.108)
  arc A2793 (52.6848, 47.108) -> (52.5832, 47.108) centre (52.634, 47.108) ccw
  arc A2794 (52.5832, 46.092) -> (52.6848, 46.092) centre (52.634, 46.092) ccw
  line L1254 (52.634, 47.108) -> (54.666, 47.108)
  arc A2795 (54.666, 47.0572) -> (54.666, 47.1588) centre (54.666, 47.108) ccw
  arc A2796 (52.634, 47.1588) -> (52.634, 47.0572) centre (52.634, 47.108) ccw
  line L1255 (54.666, 47.108) -> (54.666, 46.092)
  arc A2797 (54.6152, 46.092) -> (54.7168, 46.092) centre (54.666, 46.092) ccw
  arc A2798 (54.7168, 47.108) -> (54.6152, 47.108) centre (54.666, 47.108) ccw
  line L1256 (7.75, 34.15) -> (5.25, 34.15)
  line L1257 (48.593, 49.3892) -> (48.593, 44.4108)
  arc A2799 (48.5422, 44.4108) -> (48.6438, 44.4108) centre (48.593, 44.4108) ccw
  arc A2800 (48.6438, 49.3892) -> (48.5422, 49.3892) centre (48.593, 49.3892) ccw
  line L1258 (48.593, 44.4108) -> (46.307, 44.4108)
  arc A2801 (46.307, 44.4616) -> (46.307, 44.36) centre (46.307, 44.4108) ccw
  arc A2802 (48.593, 44.36) -> (48.593, 44.4616) centre (48.593, 44.4108) ccw
  line L1259 (46.307, 44.4108) -> (46.307, 49.3892)
  arc A2803 (46.3578, 49.3892) -> (46.2562, 49.3892) centre (46.307, 49.3892) ccw
  arc A2804 (46.2562, 44.4108) -> (46.3578, 44.4108) centre (46.307, 44.4108) ccw
  line L1260 (46.307, 49.3892) -> (48.593, 49.3892)
  arc A2805 (48.593, 49.3384) -> (48.593, 49.44) centre (48.593, 49.3892) ccw
  arc A2806 (46.307, 49.44) -> (46.307, 49.3384) centre (46.307, 49.3892) ccw
  arc A2807 (5.25, 34.1817) -> (5.25, 34.1183) centre (5.25, 34.15) ccw
  line L1261 (53.634, 45.108) -> (55.666, 45.108)
  arc A2808 (55.666, 45.0572) -> (55.666, 45.1588) centre (55.666, 45.108) ccw
  arc A2809 (53.634, 45.1588) -> (53.634, 45.0572) centre (53.634, 45.108) ccw
  line L1262 (55.666, 45.108) -> (55.666, 44.092)
  arc A2810 (55.6152, 44.092) -> (55.7168, 44.092) centre (55.666, 44.092) ccw
  arc A2811 (55.7168, 45.108) -> (55.6152, 45.108) centre (55.666, 45.108) ccw
  line L1263 (55.666, 44.092) -> (53.634, 44.092)
  arc A2812 (53.634, 44.1428) -> (53.634, 44.0412) centre (53.634, 44.092) ccw
  arc A2813 (55.666, 44.0412) -> (55.666, 44.1428) centre (55.666, 44.092) ccw
  line L1264 (53.634, 44.092) -> (53.634, 45.108)
  arc A2814 (53.6848, 45.108) -> (53.5832, 45.108) centre (53.634, 45.108) ccw
  arc A2815 (53.5832, 44.092) -> (53.6848, 44.092) centre (53.634, 44.092) ccw
  arc A2816 (7.75, 34.1183) -> (7.75, 34.1817) centre (7.75, 34.15) ccw
  line L1265 (53.634, 44.108) -> (55.666, 44.108)
  arc A2817 (55.666, 44.0572) -> (55.666, 44.1588) centre (55.666, 44.108) ccw
  arc A2818 (53.634, 44.1588) -> (53.634, 44.0572) centre (53.634, 44.108) ccw
  line L1266 (55.666, 44.108) -> (55.666, 43.092)
  arc A2819 (55.6152, 43.092) -> (55.7168, 43.092) centre (55.666, 43.092) ccw
  arc A2820 (55.7168, 44.108) -> (55.6152, 44.108) centre (55.666, 44.108) ccw
  line L1267 (55.666, 43.092) -> (53.634, 43.092)
  arc A2821 (53.634, 43.1428) -> (53.634, 43.0412) centre (53.634, 43.092) ccw
  arc A2822 (55.666, 43.0412) -> (55.666, 43.1428) centre (55.666, 43.092) ccw
  line L1268 (53.634, 43.092) -> (53.634, 44.108)
  arc A2823 (53.6848, 44.108) -> (53.5832, 44.108) centre (53.634, 44.108) ccw
  arc A2824 (53.5832, 43.092) -> (53.6848, 43.092) centre (53.634, 43.092) ccw
  arc A2825 (7.1, 34.8) -> (7.1, 35) centre (7.1, 34.9) ccw
  line L1269 (49.658, 46.116) -> (49.658, 44.084)
  arc A2826 (49.6072, 44.084) -> (49.7088, 44.084) centre (49.658, 44.084) ccw
  arc A2827 (49.7088, 46.116) -> (49.6072, 46.116) centre (49.658, 46.116) ccw
  line L1270 (49.658, 44.084) -> (48.642, 44.084)
  arc A2828 (48.642, 44.1348) -> (48.642, 44.0332) centre (48.642, 44.084) ccw
  arc A2829 (49.658, 44.0332) -> (49.658, 44.1348) centre (49.658, 44.084) ccw
  line L1271 (48.642, 44.084) -> (48.642, 46.116)
  arc A2830 (48.6928, 46.116) -> (48.5912, 46.116) centre (48.642, 46.116) ccw
  arc A2831 (48.5912, 44.084) -> (48.6928, 44.084) centre (48.642, 44.084) ccw
  line L1272 (48.642, 46.116) -> (49.658, 46.116)
  arc A2832 (49.658, 46.0652) -> (49.658, 46.1668) centre (49.658, 46.116) ccw
  arc A2833 (48.642, 46.1668) -> (48.642, 46.0652) centre (48.642, 46.116) ccw
  arc A2834 (7.1, 35) -> (7.1, 34.8) centre (7.1, 34.9) ccw
  line L1273 (58.666, 46.092) -> (56.634, 46.092)
  arc A2835 (56.634, 46.1428) -> (56.634, 46.0412) centre (56.634, 46.092) ccw
  arc A2836 (58.666, 46.0412) -> (58.666, 46.1428) centre (58.666, 46.092) ccw
  line L1274 (56.634, 46.092) -> (56.634, 47.108)
  arc A2837 (56.6848, 47.108) -> (56.5832, 47.108) centre (56.634, 47.108) ccw
  arc A2838 (56.5832, 46.092) -> (56.6848, 46.092) centre (56.634, 46.092) ccw
  line L1275 (56.634, 47.108) -> (58.666, 47.108)
  arc A2839 (58.666, 47.0572) -> (58.666, 47.1588) centre (58.666, 47.108) ccw
  arc A2840 (56.634, 47.1588) -> (56.634, 47.0572) centre (56.634, 47.108) ccw
  line L1276 (58.666, 47.108) -> (58.666, 46.092)
  arc A2841 (58.6152, 46.092) -> (58.7168, 46.092) centre (58.666, 46.092) ccw
  arc A2842 (58.7168, 47.108) -> (58.6152, 47.108) centre (58.666, 47.108) ccw
  line L1277 (48.642, 42.084) -> (48.642, 44.116)
  arc A2843 (48.6928, 44.116) -> (48.5912, 44.116) centre (48.642, 44.116) ccw
  arc A2844 (48.5912, 42.084) -> (48.6928, 42.084) centre (48.642, 42.084) ccw
  line L1278 (48.642, 44.116) -> (49.658, 44.116)
  arc A2845 (49.658, 44.0652) -> (49.658, 44.1668) centre (49.658, 44.116) ccw
  arc A2846 (48.642, 44.1668) -> (48.642, 44.0652) centre (48.642, 44.116) ccw
  line L1279 (49.658, 44.116) -> (49.658, 42.084)
  arc A2847 (49.6072, 42.084) -> (49.7088, 42.084) centre (49.658, 42.084) ccw
  arc A2848 (49.7088, 44.116) -> (49.6072, 44.116) centre (49.658, 44.116) ccw
  line L1280 (49.658, 42.084) -> (48.642, 42.084)
  arc A2849 (48.642, 42.1348) -> (48.642, 42.0332) centre (48.642, 42.084) ccw
  arc A2850 (49.658, 42.0332) -> (49.658, 42.1348) centre (49.658, 42.084) ccw
  line L1281 (48.642, 46.084) -> (48.642, 48.116)
  arc A2851 (48.6928, 48.116) -> (48.5912, 48.116) centre (48.642, 48.116) ccw
  arc A2852 (48.5912, 46.084) -> (48.6928, 46.084) centre (48.642, 46.084) ccw
  line L1282 (48.642, 48.116) -> (49.658, 48.116)
  arc A2853 (49.658, 48.0652) -> (49.658, 48.1668) centre (49.658, 48.116) ccw
  arc A2854 (48.642, 48.1668) -> (48.642, 48.0652) centre (48.642, 48.116) ccw
  line L1283 (49.658, 48.116) -> (49.658, 46.084)
  arc A2855 (49.6072, 46.084) -> (49.7088, 46.084) centre (49.658, 46.084) ccw
  arc A2856 (49.7088, 48.116) -> (49.6072, 48.116) centre (49.658, 48.116) ccw
  line L1284 (49.658, 46.084) -> (48.642, 46.084)
  arc A2857 (48.642, 46.1348) -> (48.642, 46.0332) centre (48.642, 46.084) ccw
  arc A2858 (49.658, 46.0332) -> (49.658, 46.1348) centre (49.658, 46.084) ccw
  line L1285 (54.666, 45.092) -> (52.634, 45.092)
  arc A2859 (52.634, 45.1428) -> (52.634, 45.0412) centre (52.634, 45.092) ccw
  arc A2860 (54.666, 45.0412) -> (54.666, 45.1428) centre (54.666, 45.092) ccw
  line L1286 (52.634, 45.092) -> (52.634, 46.108)
  arc A2861 (52.6848, 46.108) -> (52.5832, 46.108) centre (52.634, 46.108) ccw
  arc A2862 (52.5832, 45.092) -> (52.6848, 45.092) centre (52.634, 45.092) ccw
  line L1287 (52.634, 46.108) -> (54.666, 46.108)
  arc A2863 (54.666, 46.0572) -> (54.666, 46.1588) centre (54.666, 46.108) ccw
  arc A2864 (52.634, 46.1588) -> (52.634, 46.0572) centre (52.634, 46.108) ccw
  line L1288 (54.666, 46.108) -> (54.666, 45.092)
  arc A2865 (54.6152, 45.092) -> (54.7168, 45.092) centre (54.666, 45.092) ccw
  arc A2866 (54.7168, 46.108) -> (54.6152, 46.108) centre (54.666, 46.108) ccw
  line L1289 (57.634, 44.108) -> (59.666, 44.108)
  arc A2867 (59.666, 44.0572) -> (59.666, 44.1588) centre (59.666, 44.108) ccw
  arc A2868 (57.634, 44.1588) -> (57.634, 44.0572) centre (57.634, 44.108) ccw
  line L1290 (59.666, 44.108) -> (59.666, 43.092)
  arc A2869 (59.6152, 43.092) -> (59.7168, 43.092) centre (59.666, 43.092) ccw
  arc A2870 (59.7168, 44.108) -> (59.6152, 44.108) centre (59.666, 44.108) ccw
  line L1291 (59.666, 43.092) -> (57.634, 43.092)
  arc A2871 (57.634, 43.1428) -> (57.634, 43.0412) centre (57.634, 43.092) ccw
  arc A2872 (59.666, 43.0412) -> (59.666, 43.1428) centre (59.666, 43.092) ccw
  line L1292 (57.634, 43.092) -> (57.634, 44.108)
  arc A2873 (57.6848, 44.108) -> (57.5832, 44.108) centre (57.634, 44.108) ccw
  arc A2874 (57.5832, 43.092) -> (57.6848, 43.092) centre (57.634, 43.092) ccw
  line L1293 (49.658, 42.116) -> (49.658, 40.084)
  arc A2875 (49.6072, 40.084) -> (49.7088, 40.084) centre (49.658, 40.084) ccw
  arc A2876 (49.7088, 42.116) -> (49.6072, 42.116) centre (49.658, 42.116) ccw
  line L1294 (49.658, 40.084) -> (48.642, 40.084)
  arc A2877 (48.642, 40.1348) -> (48.642, 40.0332) centre (48.642, 40.084) ccw
  arc A2878 (49.658, 40.0332) -> (49.658, 40.1348) centre (49.658, 40.084) ccw
  line L1295 (48.642, 40.084) -> (48.642, 42.116)
  arc A2879 (48.6928, 42.116) -> (48.5912, 42.116) centre (48.642, 42.116) ccw
  arc A2880 (48.5912, 40.084) -> (48.6928, 40.084) centre (48.642, 40.084) ccw
  line L1296 (48.642, 42.116) -> (49.658, 42.116)
  arc A2881 (49.658, 42.0652) -> (49.658, 42.1668) centre (49.658, 42.116) ccw
  arc A2882 (48.642, 42.1668) -> (48.642, 42.0652) centre (48.642, 42.116) ccw
  line L1297 (54.666, 42.092) -> (52.634, 42.092)
  arc A2883 (52.634, 42.1428) -> (52.634, 42.0412) centre (52.634, 42.092) ccw
  arc A2884 (54.666, 42.0412) -> (54.666, 42.1428) centre (54.666, 42.092) ccw
  line L1298 (52.634, 42.092) -> (52.634, 43.108)
  arc A2885 (52.6848, 43.108) -> (52.5832, 43.108) centre (52.634, 43.108) ccw
  arc A2886 (52.5832, 42.092) -> (52.6848, 42.092) centre (52.634, 42.092) ccw
  line L1299 (52.634, 43.108) -> (54.666, 43.108)
  arc A2887 (54.666, 43.0572) -> (54.666, 43.1588) centre (54.666, 43.108) ccw
  arc A2888 (52.634, 43.1588) -> (52.634, 43.0572) centre (52.634, 43.108) ccw
  line L1300 (54.666, 43.108) -> (54.666, 42.092)
  arc A2889 (54.6152, 42.092) -> (54.7168, 42.092) centre (54.666, 42.092) ccw
  arc A2890 (54.7168, 43.108) -> (54.6152, 43.108) centre (54.666, 43.108) ccw
  line L1301 (58.634, 41.108) -> (60.666, 41.108)
  arc A2891 (60.666, 41.0572) -> (60.666, 41.1588) centre (60.666, 41.108) ccw
  arc A2892 (58.634, 41.1588) -> (58.634, 41.0572) centre (58.634, 41.108) ccw
  line L1302 (60.666, 41.108) -> (60.666, 40.092)
  arc A2893 (60.6152, 40.092) -> (60.7168, 40.092) centre (60.666, 40.092) ccw
  arc A2894 (60.7168, 41.108) -> (60.6152, 41.108) centre (60.666, 41.108) ccw
  line L1303 (60.666, 40.092) -> (58.634, 40.092)
  arc A2895 (58.634, 40.1428) -> (58.634, 40.0412) centre (58.634, 40.092) ccw
  arc A2896 (60.666, 40.0412) -> (60.666, 40.1428) centre (60.666, 40.092) ccw
  line L1304 (58.634, 40.092) -> (58.634, 41.108)
  arc A2897 (58.6848, 41.108) -> (58.5832, 41.108) centre (58.634, 41.108) ccw
  arc A2898 (58.5832, 40.092) -> (58.6848, 40.092) centre (58.634, 40.092) ccw
  line L1305 (57.634, 46.108) -> (59.666, 46.108)
  arc A2899 (59.666, 46.0572) -> (59.666, 46.1588) centre (59.666, 46.108) ccw
  arc A2900 (57.634, 46.1588) -> (57.634, 46.0572) centre (57.634, 46.108) ccw
  line L1306 (59.666, 46.108) -> (59.666, 45.092)
  arc A2901 (59.6152, 45.092) -> (59.7168, 45.092) centre (59.666, 45.092) ccw
  arc A2902 (59.7168, 46.108) -> (59.6152, 46.108) centre (59.666, 46.108) ccw
  line L1307 (59.666, 45.092) -> (57.634, 45.092)
  arc A2903 (57.634, 45.1428) -> (57.634, 45.0412) centre (57.634, 45.092) ccw
  arc A2904 (59.666, 45.0412) -> (59.666, 45.1428) centre (59.666, 45.092) ccw
  line L1308 (57.634, 45.092) -> (57.634, 46.108)
  arc A2905 (57.6848, 46.108) -> (57.5832, 46.108) centre (57.634, 46.108) ccw
  arc A2906 (57.5832, 45.092) -> (57.6848, 45.092) centre (57.634, 45.092) ccw
  line L1309 (58.634, 40.108) -> (60.666, 40.108)
  arc A2907 (60.666, 40.0572) -> (60.666, 40.1588) centre (60.666, 40.108) ccw
  arc A2908 (58.634, 40.1588) -> (58.634, 40.0572) centre (58.634, 40.108) ccw
  line L1310 (60.666, 40.108) -> (60.666, 39.092)
  arc A2909 (60.6152, 39.092) -> (60.7168, 39.092) centre (60.666, 39.092) ccw
  arc A2910 (60.7168, 40.108) -> (60.6152, 40.108) centre (60.666, 40.108) ccw
  line L1311 (60.666, 39.092) -> (58.634, 39.092)
  arc A2911 (58.634, 39.1428) -> (58.634, 39.0412) centre (58.634, 39.092) ccw
  arc A2912 (60.666, 39.0412) -> (60.666, 39.1428) centre (60.666, 39.092) ccw
  line L1312 (58.634, 39.092) -> (58.634, 40.108)
  arc A2913 (58.6848, 40.108) -> (58.5832, 40.108) centre (58.634, 40.108) ccw
  arc A2914 (58.5832, 39.092) -> (58.6848, 39.092) centre (58.634, 39.092) ccw
  line L1313 (59.642, 43.084) -> (59.642, 45.116)
  arc A2915 (59.6928, 45.116) -> (59.5912, 45.116) centre (59.642, 45.116) ccw
  arc A2916 (59.5912, 43.084) -> (59.6928, 43.084) centre (59.642, 43.084) ccw
  line L1314 (59.642, 45.116) -> (60.658, 45.116)
  arc A2917 (60.658, 45.0652) -> (60.658, 45.1668) centre (60.658, 45.116) ccw
  arc A2918 (59.642, 45.1668) -> (59.642, 45.0652) centre (59.642, 45.116) ccw
  line L1315 (60.658, 45.116) -> (60.658, 43.084)
  arc A2919 (60.6072, 43.084) -> (60.7088, 43.084) centre (60.658, 43.084) ccw
  arc A2920 (60.7088, 45.116) -> (60.6072, 45.116) centre (60.658, 45.116) ccw
  line L1316 (60.658, 43.084) -> (59.642, 43.084)
  arc A2921 (59.642, 43.1348) -> (59.642, 43.0332) centre (59.642, 43.084) ccw
  arc A2922 (60.658, 43.0332) -> (60.658, 43.1348) centre (60.658, 43.084) ccw
  line L1317 (57.634, 43.108) -> (59.666, 43.108)
  arc A2923 (59.666, 43.0572) -> (59.666, 43.1588) centre (59.666, 43.108) ccw
  arc A2924 (57.634, 43.1588) -> (57.634, 43.0572) centre (57.634, 43.108) ccw
  line L1318 (59.666, 43.108) -> (59.666, 42.092)
  arc A2925 (59.6152, 42.092) -> (59.7168, 42.092) centre (59.666, 42.092) ccw
  arc A2926 (59.7168, 43.108) -> (59.6152, 43.108) centre (59.666, 43.108) ccw
  line L1319 (59.666, 42.092) -> (57.634, 42.092)
  arc A2927 (57.634, 42.1428) -> (57.634, 42.0412) centre (57.634, 42.092) ccw
  arc A2928 (59.666, 42.0412) -> (59.666, 42.1428) centre (59.666, 42.092) ccw
  line L1320 (57.634, 42.092) -> (57.634, 43.108)
  arc A2929 (57.6848, 43.108) -> (57.5832, 43.108) centre (57.634, 43.108) ccw